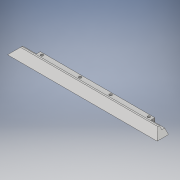
# Autodesk Inventor part: PlogPiramida
Saved by Autodesk Inventor 2019 (Build 230136000, 136)
## iProperties
Created: 2022-02-07
Part Number: PlogPiramida
Material: Ogólny
Document SubType Name: Modeling
Designer: Michał
Density: 1 g/cm^3
Appearance: Domyślna
Author: Michał
Autodesk Inventor part; units mm, degrees
ref_plane "YZ Plane" through (0, 0, 0) normal (1, 0, 0) x (0, 1, 0)
ref_plane "XZ Plane" through (0, 0, 0) normal (0, 1, 0) x (-1, 0, 0)
ref_plane "XY Plane" through (0, 0, 0) normal (0, 0, 1) x (1, 0, 0)
sketch "Szkic1" plane through (0, 0, 0) normal (1, 0, 0) x (0, 1, 0)
  line L0 (0, 0) -> (0, -20.1)
  line L1 (0, -20.1) -> (8, -20.1)
  line L2 (8, -20.1) -> (8, -9)
  line L3 (8, -9) -> (0, 0)
  line L4 (8, -20.1) -> (5, -20.1)
  line L5 (5, -20.1) -> (5, -11)
  line L6 (5, -11) -> (8, -11)
  line L7 (8, -11) -> (8, -20.1)
  line L8 (5, -14.9) -> (0, -14.9)
  dimension "d0" = 20.1
  dimension "d2" = 8
  dimension "d4" = 3
  dimension "d5" = 5.2
  dimension "d25" = 11
  dimension "d26" = 2
  constraints: 18 end point, 4 perpendicular, 2 parallel, 2 point on line, 1 horizontal, 1 vertical
  measures "d0" distance of L0.start L0.end
  measures "d2" distance of L0.end L1.end
  measures "d4" distance of L5.end L6.end
  measures "d5" distance between parallel lines of L1 L8
  measures "d25" distance from line of L0.start L6
  measures "d26" distance from line of L2.end L6
extrude "Wyciągnięcie proste1" add sketch "Szkic1" along normal mid plane 196 contours L3 L2 L6 L5 L8 L0
extrude "Wyciągnięcie proste2" add sketch "Szkic1" along normal mid plane 150 contours L8 L5 L1 L0
sketch "Szkic3" plane through (-98, 0, 0) normal (0, -1, 0) x (1, 0, 0)
  line L0 (98, 0) -> (98, -20.1) construction
  line L1 (23, -20.1) -> (173, -20.1) construction
  point P0 (168, -17.1)
  point P1 (118, -17.1)
  point P2 (28, -17.1)
  point P3 (78, -17.1)
  dimension "d12" = 20
  dimension "d13" = 70
  dimension "d14" = 3
  constraints: 2 end point, 2 symmetric about line, 1 horizontal alignment, 1 midpoint
  measures "d12" distance from line of L0 point (118, -17.1)
  measures "d13" distance from line of L0 point (168, -17.1)
  measures "d14" distance from line of L1 point (168, -17.1)
hole "Otwór1" at (70, 0, -17.1) at (20, 0, -17.1) at (-20, 0, -17.1) at (-70, 0, -17.1) direction (0, 1, 0) diameter 3.4 end through all countersink diameter 6.9 countersink angle 84.225 clearance for "Śruba ze łbem stożkowym ISO 2009/7046" size "M3" standard "ISO"
sketch "Szkic4" plane through (75, 5, -20.1) normal (0, 0, -1) x (-1, 0, 0)
  line L0 (-23, 3) -> (-23, -5) projected
  line L1 (-23, -5) -> (-15, 3)
  line L2 (-23, 3) -> (173, 3) construction
  line L3 (-23, 3) -> (-23, -5)
  line L4 (-23, -5) -> (173, -5) construction
  line L5 (173, -5) -> (173, 3)
  line L6 (173, 3) -> (165, 3)
  line L7 (165, 3) -> (173, -5)
  line L8 (-23, 3) -> (-15, 3)
  point P0 (75, -5)
  dimension "d22" = 45
  constraints: 12 end point, 2 perpendicular, 2 vertical, 1 collinear, 1 point on line
  measures "d22" angle of L5 L7
extrude "Wyciągnięcie proste3" cut sketch "Szkic4" against normal through all
